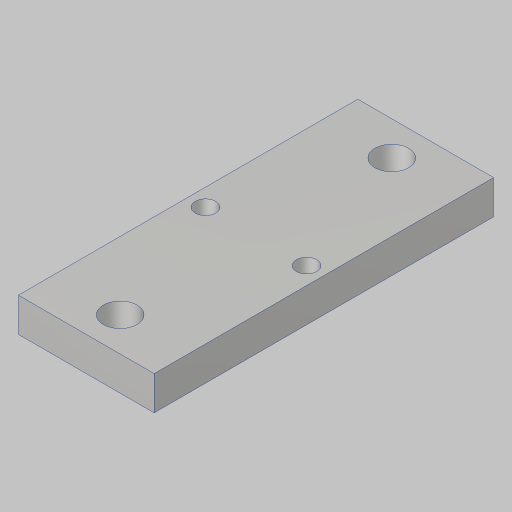
# Autodesk Inventor part: DB1-010
Saved by Autodesk Inventor 2023.5 (Build 275446000, 446)
## iProperties
Created: 2025-01-31
Part Number: DB1-010
Material: Aluminum 6061
Document SubType Name: Modeling
Designer: slick
Density: 2.7 g/cm^3
Appearance: Aluminum - Flat
Author: slick
Autodesk Inventor part; units mm, degrees
ref_plane "YZ Plane" through (0, 0, 0) normal (1, 0, 0) x (0, 1, 0)
ref_plane "XZ Plane" through (0, 0, 0) normal (0, 1, 0) x (-1, 0, 0)
ref_plane "XY Plane" through (0, 0, 0) normal (0, 0, 1) x (1, 0, 0)
sketch "Sketch1" plane through (0, 0, 0) normal (0, 1, 0) x (-1, 0, 0)
  line L0 (-12.7, -31.75) -> (12.7, -31.75)
  line L1 (12.7, -31.75) -> (12.7, 31.75)
  line L2 (12.7, 31.75) -> (-12.7, 31.75)
  line L3 (-12.7, 31.75) -> (-12.7, -31.75)
  line L4 (-12.7, -31.75) -> (12.7, 31.75) construction
  line L5 (12.7, -31.75) -> (-12.7, 31.75) construction
  point P0 (0, 0)
  dimension "d0" = 25.4
  dimension "d1" = 63.5
  constraints: 12 end point, 2 midpoint, 2 parallel, 1 horizontal, 1 perpendicular
  measures "d0" distance of L1.end L2.end
  measures "d1" distance of L0.end L1.end
extrude "Extrusion1" add sketch "Sketch1" along normal blind 6.35
sketch "Sketch2" plane through (0, 6.35, 0) normal (0, 1, 0) x (1, 0, 0)
  line L0 (0, -25.4) -> (0, 25.4) construction
  line L1 (-12.7, 31.75) -> (-12.7, -31.75) construction
  point P0 (0, 0)
  point P1 (0, 0)
  dimension "d4" = 50.8
  constraints: 2 end point, 2 vertical alignment, 1 coincident, 1 midpoint, 1 vertical
  measures "d4" distance of L0.start L0.end
hole "Hole1" at (0, 6.35, 25.4) at (0, 6.35, -25.4) direction (0, -1, 0) diameter 6.3 end through all
sketch "Sketch3" plane through (0, 6.35, 0) normal (0, 1, 0) x (1, 0, 0)
  line L0 (-9.4578, 0) -> (9.4578, 0) construction
  point P0 (0, 0)
  point P1 (0, 0)
  dimension "d13" = 18.9155
  constraints: 2 end point, 2 horizontal alignment, 1 coincident, 1 horizontal, 1 midpoint
  measures "d13" distance of L0.start L0.end
hole "Hole2" at (-9.4578, 6.35, 0) at (9.4578, 6.35, 0) direction (0, -1, 0) diameter 3.81 end through all clearance for "Flat Head Machine Screw (82)" size "#6" standard "Ansi Unified Screw Threads"
body "Solid1"
